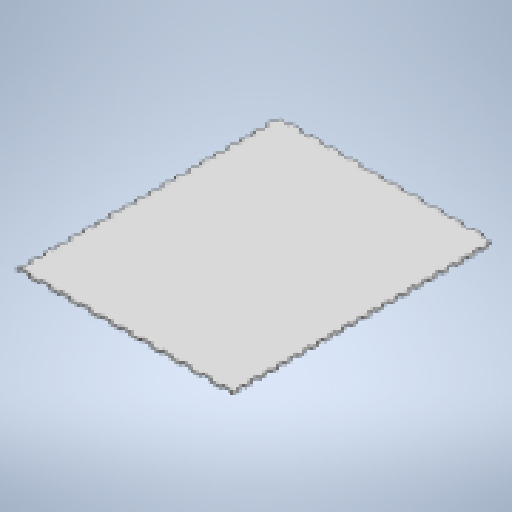
# Autodesk Inventor part: BaseBoard
Saved by Autodesk Inventor 2024 (Build 280153000, 153)
## iProperties
Created: 2023-09-08
Part Number: BaseBoard
Material: Generic
Document SubType Name: Modeling
Designer: Bruno
Density: 1 g/cm^3
Appearance: Default
Author: Bruno
Autodesk Inventor part; units mm, degrees
ref_plane "YZ Plane" through (0, 0, 0) normal (1, 0, 0) x (0, 1, 0)
ref_plane "XZ Plane" through (0, 0, 0) normal (0, 1, 0) x (-1, 0, 0)
ref_plane "XY Plane" through (0, 0, 0) normal (0, 0, 1) x (1, 0, 0)
sketch "Sketch1" plane through (0, 0, 0) normal (0, 1, 0) x (-1, 0, 0)
  line L0 (159.0322, -235.7679) -> (159.0322, 129.2321) projected
  line L1 (159.0322, 129.2321) -> (-140.9678, 129.2321) projected
  line L2 (-140.9678, 129.2321) -> (-140.9678, -235.7679) projected
  line L3 (-140.9678, -235.7679) -> (159.0322, -235.7679) projected
  line L4 (159.0322, -226.6429) -> (159.0322, -235.7679) projected
  line L5 (159.0322, -235.7679) -> (156.0322, -235.7679) projected
  line L6 (156.0322, -226.6429) -> (156.0322, -235.7679) projected
  line L7 (159.0322, -226.6429) -> (156.0322, -226.6429) projected
  line L8 (159.0322, -208.3929) -> (159.0322, -217.5179) projected
  line L9 (159.0322, -217.5179) -> (156.0322, -217.5179) projected
  line L10 (156.0322, -208.3929) -> (156.0322, -217.5179) projected
  line L11 (159.0322, -208.3929) -> (156.0322, -208.3929) projected
  line L12 (159.0322, -190.1429) -> (159.0322, -199.2679) projected
  line L13 (159.0322, -199.2679) -> (156.0322, -199.2679) projected
  line L14 (156.0322, -190.1429) -> (156.0322, -199.2679) projected
  line L15 (159.0322, -190.1429) -> (156.0322, -190.1429) projected
  line L16 (159.0322, -171.8929) -> (159.0322, -181.0179) projected
  line L17 (159.0322, -181.0179) -> (156.0322, -181.0179) projected
  line L18 (156.0322, -171.8929) -> (156.0322, -181.0179) projected
  line L19 (159.0322, -171.8929) -> (156.0322, -171.8929) projected
  line L20 (159.0322, -153.6429) -> (159.0322, -162.7679) projected
  line L21 (159.0322, -162.7679) -> (156.0322, -162.7679) projected
  line L22 (156.0322, -153.6429) -> (156.0322, -162.7679) projected
  line L23 (159.0322, -153.6429) -> (156.0322, -153.6429) projected
  line L24 (159.0322, -135.3929) -> (159.0322, -144.5179) projected
  line L25 (159.0322, -144.5179) -> (156.0322, -144.5179) projected
  line L26 (156.0322, -135.3929) -> (156.0322, -144.5179) projected
  line L27 (159.0322, -135.3929) -> (156.0322, -135.3929) projected
  line L28 (159.0322, -117.1429) -> (159.0322, -126.2679) projected
  line L29 (159.0322, -126.2679) -> (156.0322, -126.2679) projected
  line L30 (156.0322, -117.1429) -> (156.0322, -126.2679) projected
  line L31 (159.0322, -117.1429) -> (156.0322, -117.1429) projected
  line L32 (159.0322, -98.8929) -> (159.0322, -108.0179) projected
  line L33 (159.0322, -108.0179) -> (156.0322, -108.0179) projected
  line L34 (156.0322, -98.8929) -> (156.0322, -108.0179) projected
  line L35 (159.0322, -98.8929) -> (156.0322, -98.8929) projected
  line L36 (159.0322, -80.6429) -> (159.0322, -89.7679) projected
  line L37 (159.0322, -80.6429) -> (159.0322, -89.7679) projected
  line L38 (159.0322, -89.7679) -> (156.0322, -89.7679) projected
  line L39 (156.0322, -80.6429) -> (156.0322, -89.7679) projected
  line L40 (159.0322, -80.6429) -> (156.0322, -80.6429) projected
  line L41 (159.0322, -62.3929) -> (159.0322, -71.5179) projected
  line L42 (159.0322, -71.5179) -> (156.0322, -71.5179) projected
  line L43 (156.0322, -62.3929) -> (156.0322, -71.5179) projected
  line L44 (159.0322, -62.3929) -> (156.0322, -62.3929) projected
  line L45 (159.0322, -44.1429) -> (159.0322, -53.2679) projected
  line L46 (159.0322, -53.2679) -> (156.0322, -53.2679) projected
  line L47 (156.0322, -44.1429) -> (156.0322, -53.2679) projected
  line L48 (159.0322, -44.1429) -> (156.0322, -44.1429) projected
  line L49 (159.0322, -25.8929) -> (159.0322, -35.0179) projected
  line L50 (159.0322, -35.0179) -> (156.0322, -35.0179) projected
  line L51 (156.0322, -25.8929) -> (156.0322, -35.0179) projected
  line L52 (159.0322, -25.8929) -> (156.0322, -25.8929) projected
  line L53 (159.0322, -7.6429) -> (159.0322, -16.7679) projected
  line L54 (159.0322, -16.7679) -> (156.0322, -16.7679) projected
  line L55 (156.0322, -7.6429) -> (156.0322, -16.7679) projected
  line L56 (159.0322, -7.6429) -> (156.0322, -7.6429) projected
  line L57 (159.0322, 10.6071) -> (159.0322, 1.4821) projected
  line L58 (159.0322, 1.4821) -> (156.0322, 1.4821) projected
  line L59 (156.0322, 10.6071) -> (156.0322, 1.4821) projected
  line L60 (159.0322, 10.6071) -> (156.0322, 10.6071) projected
  line L61 (159.0322, 28.8571) -> (159.0322, 19.7321) projected
  line L62 (159.0322, 19.7321) -> (156.0322, 19.7321) projected
  line L63 (156.0322, 28.8571) -> (156.0322, 19.7321) projected
  line L64 (159.0322, 28.8571) -> (156.0322, 28.8571) projected
  line L65 (159.0322, 47.1071) -> (159.0322, 37.9821) projected
  line L66 (159.0322, 37.9821) -> (156.0322, 37.9821) projected
  line L67 (156.0322, 47.1071) -> (156.0322, 37.9821) projected
  line L68 (159.0322, 47.1071) -> (156.0322, 47.1071) projected
  line L69 (159.0322, 65.3571) -> (159.0322, 56.2321) projected
  line L70 (159.0322, 56.2321) -> (156.0322, 56.2321) projected
  line L71 (156.0322, 65.3571) -> (156.0322, 56.2321) projected
  line L72 (159.0322, 65.3571) -> (156.0322, 65.3571) projected
  line L73 (159.0322, 83.6071) -> (159.0322, 74.4821) projected
  line L74 (159.0322, 74.4821) -> (156.0322, 74.4821) projected
  line L75 (156.0322, 83.6071) -> (156.0322, 74.4821) projected
  line L76 (159.0322, 83.6071) -> (156.0322, 83.6071) projected
  line L77 (159.0322, 101.8571) -> (159.0322, 92.7321) projected
  line L78 (159.0322, 92.7321) -> (156.0322, 92.7321) projected
  line L79 (156.0322, 101.8571) -> (156.0322, 92.7321) projected
  line L80 (159.0322, 101.8571) -> (156.0322, 101.8571) projected
  line L81 (159.0322, 120.1071) -> (159.0322, 110.9821) projected
  line L82 (159.0322, 110.9821) -> (156.0322, 110.9821) projected
  line L83 (156.0322, 120.1071) -> (156.0322, 110.9821) projected
  line L84 (159.0322, 120.1071) -> (156.0322, 120.1071) projected
  line L85 (142.0322, -232.7679) -> (156.0322, -232.7679) projected
  line L86 (156.0322, -232.7679) -> (156.0322, -235.7679) projected
  line L87 (142.0322, -235.7679) -> (156.0322, -235.7679) projected
  line L88 (142.0322, -232.7679) -> (142.0322, -235.7679) projected
  line L89 (114.0322, -232.7679) -> (128.0322, -232.7679) projected
  line L90 (128.0322, -232.7679) -> (128.0322, -235.7679) projected
  line L91 (114.0322, -235.7679) -> (128.0322, -235.7679) projected
  line L92 (114.0322, -232.7679) -> (114.0322, -235.7679) projected
  line L93 (86.0322, -232.7679) -> (100.0322, -232.7679) projected
  line L94 (100.0322, -232.7679) -> (100.0322, -235.7679) projected
  line L95 (86.0322, -235.7679) -> (100.0322, -235.7679) projected
  line L96 (86.0322, -232.7679) -> (86.0322, -235.7679) projected
  line L97 (58.0322, -232.7679) -> (72.0322, -232.7679) projected
  line L98 (72.0322, -232.7679) -> (72.0322, -235.7679) projected
  line L99 (58.0322, -235.7679) -> (72.0322, -235.7679) projected
  line L100 (58.0322, -232.7679) -> (58.0322, -235.7679) projected
  line L101 (30.0322, -232.7679) -> (44.0322, -232.7679) projected
  line L102 (44.0322, -232.7679) -> (44.0322, -235.7679) projected
  line L103 (30.0322, -235.7679) -> (44.0322, -235.7679) projected
  line L104 (30.0322, -232.7679) -> (30.0322, -235.7679) projected
  line L105 (2.0322, -232.7679) -> (16.0322, -232.7679) projected
  line L106 (16.0322, -232.7679) -> (16.0322, -235.7679) projected
  line L107 (2.0322, -235.7679) -> (16.0322, -235.7679) projected
  line L108 (2.0322, -232.7679) -> (2.0322, -235.7679) projected
  line L109 (-25.9678, -232.7679) -> (-11.9678, -232.7679) projected
  line L110 (-11.9678, -232.7679) -> (-11.9678, -235.7679) projected
  line L111 (-25.9678, -235.7679) -> (-11.9678, -235.7679) projected
  line L112 (-25.9678, -232.7679) -> (-25.9678, -235.7679) projected
  line L113 (-53.9678, -232.7679) -> (-39.9678, -232.7679) projected
  line L114 (-39.9678, -232.7679) -> (-39.9678, -235.7679) projected
  line L115 (-53.9678, -235.7679) -> (-39.9678, -235.7679) projected
  line L116 (-53.9678, -232.7679) -> (-53.9678, -235.7679) projected
  line L117 (-81.9678, -232.7679) -> (-67.9678, -232.7679) projected
  line L118 (-67.9678, -232.7679) -> (-67.9678, -235.7679) projected
  line L119 (-81.9678, -235.7679) -> (-67.9678, -235.7679) projected
  line L120 (-81.9678, -232.7679) -> (-81.9678, -235.7679) projected
  line L121 (-109.9678, -232.7679) -> (-95.9678, -232.7679) projected
  line L122 (-95.9678, -232.7679) -> (-95.9678, -235.7679) projected
  line L123 (-109.9678, -235.7679) -> (-95.9678, -235.7679) projected
  line L124 (-109.9678, -232.7679) -> (-109.9678, -235.7679) projected
  line L125 (-137.9678, -232.7679) -> (-123.9678, -232.7679) projected
  line L126 (-123.9678, -232.7679) -> (-123.9678, -235.7679) projected
  line L127 (-137.9678, -235.7679) -> (-123.9678, -235.7679) projected
  line L128 (-137.9678, -232.7679) -> (-137.9678, -235.7679) projected
  line L129 (-137.9678, -226.6429) -> (-137.9678, -235.7679) projected
  line L130 (-137.9678, -235.7679) -> (-140.9678, -235.7679) projected
  line L131 (-140.9678, -226.6429) -> (-140.9678, -235.7679) projected
  line L132 (-137.9678, -226.6429) -> (-140.9678, -226.6429) projected
  line L133 (-137.9678, -208.3929) -> (-137.9678, -217.5179) projected
  line L134 (-137.9678, -217.5179) -> (-140.9678, -217.5179) projected
  line L135 (-140.9678, -208.3929) -> (-140.9678, -217.5179) projected
  line L136 (-137.9678, -208.3929) -> (-140.9678, -208.3929) projected
  line L137 (-137.9678, -190.1429) -> (-137.9678, -199.2679) projected
  line L138 (-137.9678, -199.2679) -> (-140.9678, -199.2679) projected
  line L139 (-140.9678, -190.1429) -> (-140.9678, -199.2679) projected
  line L140 (-137.9678, -190.1429) -> (-140.9678, -190.1429) projected
  line L141 (-137.9678, -171.8929) -> (-137.9678, -181.0179) projected
  line L142 (-137.9678, -181.0179) -> (-140.9678, -181.0179) projected
  line L143 (-140.9678, -171.8929) -> (-140.9678, -181.0179) projected
  line L144 (-137.9678, -171.8929) -> (-140.9678, -171.8929) projected
  line L145 (-137.9678, -153.6429) -> (-137.9678, -162.7679) projected
  line L146 (-137.9678, -162.7679) -> (-140.9678, -162.7679) projected
  line L147 (-140.9678, -153.6429) -> (-140.9678, -162.7679) projected
  line L148 (-137.9678, -153.6429) -> (-140.9678, -153.6429) projected
  line L149 (-137.9678, -135.3929) -> (-137.9678, -144.5179) projected
  line L150 (-137.9678, -144.5179) -> (-140.9678, -144.5179) projected
  line L151 (-140.9678, -135.3929) -> (-140.9678, -144.5179) projected
  line L152 (-137.9678, -135.3929) -> (-140.9678, -135.3929) projected
  line L153 (-137.9678, -117.1429) -> (-137.9678, -126.2679) projected
  line L154 (-137.9678, -126.2679) -> (-140.9678, -126.2679) projected
  line L155 (-140.9678, -117.1429) -> (-140.9678, -126.2679) projected
  line L156 (-137.9678, -117.1429) -> (-140.9678, -117.1429) projected
  line L157 (-137.9678, -98.8929) -> (-137.9678, -108.0179) projected
  line L158 (-137.9678, -108.0179) -> (-140.9678, -108.0179) projected
  line L159 (-140.9678, -98.8929) -> (-140.9678, -108.0179) projected
  line L160 (-137.9678, -98.8929) -> (-140.9678, -98.8929) projected
  line L161 (-137.9678, -80.6429) -> (-137.9678, -89.7679) projected
  line L162 (-137.9678, -89.7679) -> (-140.9678, -89.7679) projected
  line L163 (-140.9678, -80.6429) -> (-140.9678, -89.7679) projected
  line L164 (-137.9678, -80.6429) -> (-140.9678, -80.6429) projected
  line L165 (-137.9678, -62.3929) -> (-137.9678, -71.5179) projected
  line L166 (-137.9678, -71.5179) -> (-140.9678, -71.5179) projected
  line L167 (-140.9678, -62.3929) -> (-140.9678, -71.5179) projected
  line L168 (-137.9678, -62.3929) -> (-140.9678, -62.3929) projected
  line L169 (-137.9678, -44.1429) -> (-137.9678, -53.2679) projected
  line L170 (-137.9678, -53.2679) -> (-140.9678, -53.2679) projected
  line L171 (-140.9678, -44.1429) -> (-140.9678, -53.2679) projected
  line L172 (-137.9678, -44.1429) -> (-140.9678, -44.1429) projected
  line L173 (-137.9678, -25.8929) -> (-137.9678, -35.0179) projected
  line L174 (-137.9678, -35.0179) -> (-140.9678, -35.0179) projected
  line L175 (-140.9678, -25.8929) -> (-140.9678, -35.0179) projected
  line L176 (-137.9678, -25.8929) -> (-140.9678, -25.8929) projected
  line L177 (-137.9678, -7.6429) -> (-137.9678, -16.7679) projected
  line L178 (-137.9678, -16.7679) -> (-140.9678, -16.7679) projected
  line L179 (-140.9678, -7.6429) -> (-140.9678, -16.7679) projected
  line L180 (-137.9678, -7.6429) -> (-140.9678, -7.6429) projected
  line L181 (-137.9678, 10.6071) -> (-137.9678, 1.4821) projected
  line L182 (-137.9678, 1.4821) -> (-140.9678, 1.4821) projected
  line L183 (-140.9678, 10.6071) -> (-140.9678, 1.4821) projected
  line L184 (-137.9678, 10.6071) -> (-140.9678, 10.6071) projected
  line L185 (-137.9678, 28.8571) -> (-137.9678, 19.7321) projected
  line L186 (-137.9678, 19.7321) -> (-140.9678, 19.7321) projected
  line L187 (-140.9678, 28.8571) -> (-140.9678, 19.7321) projected
  line L188 (-137.9678, 28.8571) -> (-140.9678, 28.8571) projected
  line L189 (-137.9678, 47.1071) -> (-137.9678, 37.9821) projected
  line L190 (-137.9678, 37.9821) -> (-140.9678, 37.9821) projected
  line L191 (-140.9678, 47.1071) -> (-140.9678, 37.9821) projected
  line L192 (-137.9678, 47.1071) -> (-140.9678, 47.1071) projected
  line L193 (-137.9678, 65.3571) -> (-137.9678, 56.2321) projected
  line L194 (-137.9678, 56.2321) -> (-140.9678, 56.2321) projected
  line L195 (-140.9678, 65.3571) -> (-140.9678, 56.2321) projected
  line L196 (-137.9678, 65.3571) -> (-140.9678, 65.3571) projected
  line L197 (-137.9678, 83.6071) -> (-137.9678, 74.4821) projected
  line L198 (-137.9678, 74.4821) -> (-140.9678, 74.4821) projected
  line L199 (-140.9678, 83.6071) -> (-140.9678, 74.4821) projected
  line L200 (-137.9678, 83.6071) -> (-140.9678, 83.6071) projected
  line L201 (-137.9678, 101.8571) -> (-137.9678, 92.7321) projected
  line L202 (-137.9678, 92.7321) -> (-140.9678, 92.7321) projected
  line L203 (-140.9678, 101.8571) -> (-140.9678, 92.7321) projected
  line L204 (-137.9678, 101.8571) -> (-140.9678, 101.8571) projected
  line L205 (-137.9678, 120.1071) -> (-137.9678, 110.9821) projected
  line L206 (-137.9678, 110.9821) -> (-140.9678, 110.9821) projected
  line L207 (-140.9678, 120.1071) -> (-140.9678, 110.9821) projected
  line L208 (-137.9678, 120.1071) -> (-140.9678, 120.1071) projected
  line L209 (-137.9678, 129.2321) -> (-123.9678, 129.2321) projected
  line L210 (-123.9678, 129.2321) -> (-123.9678, 126.2321) projected
  line L211 (-137.9678, 126.2321) -> (-123.9678, 126.2321) projected
  line L212 (-137.9678, 129.2321) -> (-137.9678, 126.2321) projected
  line L213 (-109.9678, 129.2321) -> (-95.9678, 129.2321) projected
  line L214 (-95.9678, 129.2321) -> (-95.9678, 126.2321) projected
  line L215 (-109.9678, 126.2321) -> (-95.9678, 126.2321) projected
  line L216 (-109.9678, 129.2321) -> (-109.9678, 126.2321) projected
  line L217 (-81.9678, 129.2321) -> (-67.9678, 129.2321) projected
  line L218 (-67.9678, 129.2321) -> (-67.9678, 126.2321) projected
  line L219 (-81.9678, 126.2321) -> (-67.9678, 126.2321) projected
  line L220 (-81.9678, 129.2321) -> (-81.9678, 126.2321) projected
  line L221 (-53.9678, 129.2321) -> (-39.9678, 129.2321) projected
  line L222 (-39.9678, 129.2321) -> (-39.9678, 126.2321) projected
  line L223 (-53.9678, 126.2321) -> (-39.9678, 126.2321) projected
  line L224 (-53.9678, 129.2321) -> (-53.9678, 126.2321) projected
  line L225 (-25.9678, 129.2321) -> (-11.9678, 129.2321) projected
  line L226 (-11.9678, 129.2321) -> (-11.9678, 126.2321) projected
  line L227 (-25.9678, 126.2321) -> (-11.9678, 126.2321) projected
  line L228 (-25.9678, 129.2321) -> (-25.9678, 126.2321) projected
  line L229 (2.0322, 129.2321) -> (16.0322, 129.2321) projected
  line L230 (16.0322, 129.2321) -> (16.0322, 126.2321) projected
  line L231 (2.0322, 126.2321) -> (16.0322, 126.2321) projected
  line L232 (2.0322, 129.2321) -> (2.0322, 126.2321) projected
  line L233 (30.0322, 129.2321) -> (44.0322, 129.2321) projected
  line L234 (44.0322, 129.2321) -> (44.0322, 126.2321) projected
  line L235 (30.0322, 126.2321) -> (44.0322, 126.2321) projected
  line L236 (30.0322, 129.2321) -> (30.0322, 126.2321) projected
  line L237 (58.0322, 129.2321) -> (72.0322, 129.2321) projected
  line L238 (72.0322, 129.2321) -> (72.0322, 126.2321) projected
  line L239 (58.0322, 126.2321) -> (72.0322, 126.2321) projected
  line L240 (58.0322, 129.2321) -> (58.0322, 126.2321) projected
  line L241 (86.0322, 129.2321) -> (100.0322, 129.2321) projected
  line L242 (100.0322, 129.2321) -> (100.0322, 126.2321) projected
  line L243 (86.0322, 126.2321) -> (100.0322, 126.2321) projected
  line L244 (86.0322, 129.2321) -> (86.0322, 126.2321) projected
  line L245 (114.0322, 129.2321) -> (128.0322, 129.2321) projected
  line L246 (128.0322, 129.2321) -> (128.0322, 126.2321) projected
  line L247 (114.0322, 126.2321) -> (128.0322, 126.2321) projected
  line L248 (114.0322, 129.2321) -> (114.0322, 126.2321) projected
  line L249 (142.0322, 129.2321) -> (156.0322, 129.2321) projected
  line L250 (156.0322, 129.2321) -> (156.0322, 126.2321) projected
  line L251 (142.0322, 126.2321) -> (156.0322, 126.2321) projected
  line L252 (142.0322, 129.2321) -> (142.0322, 126.2321) projected
  point P0 (0, 0)
  constraints: 4 other
extrude "Extrusion1" add sketch "Sketch1" along normal blind 3 contours L7 L6 L85 L88 L3 L90 L89 L92 L94 L93 L96 L98 L97 L100 L102 L101 L104 L106 L105 L108 L110 L109 L112 L114 L113 L116 L118 L117 L120 L122 L121 L124 L126 L125 L129 L132 L2 L134 L133 L136 L138 L137 L140 L142 L141 L144 L146 L145 L148 L150 L149 L152 L154 L153 L156 L158 L157 L160 L162 L161 L164 L166 L165 L168 L170 L169 L172 L174 L173 L176 L178 L177 L180 L182 L181 L184 L186 L185 L188 L190 L189 L192 L194 L193 L196 L198 L197 L200 L202 L201 L204 L206 L205 L208 L1 L212 L211 L210 L216 L215 L214 L220 L219 L218 L224 L223 L222 L228 L227 L226 L232 L231 L230 L236 L235 L234 L240 L239 L238 L244 L243 L242 L248 L247 L246 L252 L251 L250 L0 L84 L83 L82 L80 L79 L78 L76 L75 L74 L72 L71 L70 L68 L67 L66 L64 L63 L62 L60 L59 L58 L56 L55 L54 L52 L51 L50 L48 L47 L46 L44 L43 L42 L40 L39 L38 L35 L34 L33 L31 L30 L29 L27 L26 L25 L23 L22 L21 L19 L18 L17 L15 L14 L13 L11 L10 L9
body "Solid1"
